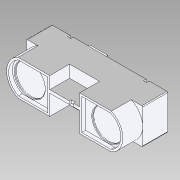
# Autodesk Inventor part: Sharp_2Y0A710
Saved by Autodesk Inventor 2017 (Build 210142000, 142)
## iProperties
Created: 2015-09-16
Part Number: Sharp_2Y0A710
Material: Generic
Document SubType Name: Modeling
Designer: JonathanC
Density: 1 g/cm^3
Appearance: PTFE
Author: JonathanC
Autodesk Inventor part; units mm, degrees
ref_plane "YZ Plane" through (0, 0, 0) normal (1, 0, 0) x (0, 1, 0)
ref_plane "XZ Plane" through (0, 0, 0) normal (0, 1, 0) x (-1, 0, 0)
ref_plane "XY Plane" through (0, 0, 0) normal (0, 0, 1) x (1, 0, 0)
sketch "Sketch1" plane through (0, 0, 0) normal (0, 0, 1) x (1, 0, 0)
  line L0 (0, 0) -> (58.039, 0)
  line L1 (58.039, 0) -> (58.039, 17.653)
  line L2 (58.039, 17.653) -> (0, 17.653)
  line L3 (0, 17.653) -> (0, 0)
  dimension "d0" = 58.039
  dimension "d1" = 17.653
  constraints: 8 end point, 2 parallel, 1 horizontal, 1 perpendicular
  measures "d0" distance of L2.end L1.end
  measures "d1" distance of L1.end L0.end
extrude "Extrusion1" add sketch "Sketch1" along normal blind 12.573
sketch "Sketch2" plane through (0, 0, 0) normal (0, 0, -1) x (-1, 0, 0)
  line L0 (0, 0) -> (-58.039, 0) projected
  line L1 (0, 17.653) -> (0, 0) projected
  line L2 (-58.039, 17.653) -> (0, 17.653) projected
  line L3 (-58.039, 0) -> (-58.039, 17.653) projected
  line L4 (-0.889, 16.764) -> (-0.889, 0.889)
  line L5 (-0.889, 0.889) -> (-57.15, 0.889)
  line L6 (-57.15, 0.889) -> (-57.15, 16.764)
  line L7 (-57.15, 16.764) -> (-0.889, 16.764)
  dimension "d4" = 0.889
  constraints: 8 end point, 3 other
  measures "d4" distance between parallel lines of L2 L7
extrude "Extrusion2" cut sketch "Sketch2" against normal blind 1.778 contours L4 L5 L6 L7
sketch "Sketch3" plane through (0, 0, 0) normal (0, -1, 0) x (1, 0, 0)
  line L0 (0, 0) -> (58.039, 0) projected
  line L1 (58.039, 0) -> (58.039, 12.573) projected
  line L2 (0, 12.573) -> (58.039, 12.573) projected
  line L3 (0, 0) -> (0, 12.573) projected
  line L4 (0, 0) -> (58.039, 0) projected
  line L5 (48.768, 0) -> (47.244, 0)
  line L6 (47.244, 0) -> (47.244, 1.27)
  line L7 (47.244, 1.27) -> (48.768, 1.27)
  line L8 (48.768, 1.27) -> (48.768, 0)
  line L9 (10.795, 0) -> (9.271, 0)
  line L10 (9.271, 0) -> (9.271, 1.27)
  line L11 (9.271, 1.27) -> (10.795, 1.27)
  line L12 (10.795, 1.27) -> (10.795, 0)
  dimension "d7" = 1.524
  dimension "d8" = 1.524
  dimension "d9" = 9.271
  dimension "d10" = 9.271
  dimension "d11" = 1.27
  dimension "d12" = 1.27
  constraints: 16 end point, 4 parallel, 2 horizontal, 2 perpendicular, 2 point on line
  measures "d7" distance of L6.end L7.end
  measures "d8" distance of L10.end L11.end
  measures "d9" distance between parallel lines of L1 L8
  measures "d10" distance between parallel lines of L3 L10
  measures "d11" distance of L11.end L9.start
  measures "d12" distance of L5.end L6.end
extrude "Extrusion3" cut sketch "Sketch3" against normal through all contours L10 L11 L12 L0 | L6 L7 L8 L0
sketch "Sketch4" plane through (0, 0, 12.573) normal (0, 0, 1) x (1, 0, 0)
  line L0 (58.039, 17.653) -> (0, 17.653) projected
  line L1 (0, 0) -> (58.039, 0) projected
  line L2 (5.715, 17.653) -> (21.59, 17.653)
  line L3 (21.59, 17.653) -> (21.59, 0)
  line L4 (21.59, 0) -> (5.715, 0)
  line L5 (5.715, 0) -> (5.715, 17.653)
  line L6 (36.5125, 17.653) -> (52.3875, 17.653)
  line L7 (52.3875, 17.653) -> (52.3875, 0)
  line L8 (52.3875, 0) -> (36.5125, 0)
  line L9 (36.5125, 0) -> (36.5125, 17.653)
  arc A0 (52.3875, 0) -> (52.3875, 17.653) centre (48.429, 8.8265) ccw
  arc A1 (5.715, 17.653) -> (5.715, 0) centre (9.6735, 8.8265) ccw
  line L10 (0, 17.653) -> (0, 0) projected
  line L11 (21.59, 11.557) -> (36.5125, 11.557)
  line L12 (36.5125, 11.557) -> (36.5125, 10.033)
  line L13 (36.5125, 10.033) -> (21.59, 10.033)
  line L14 (21.59, 10.033) -> (21.59, 11.557)
  dimension "d17" = 15.875
  dimension "d18" = 15.875
  dimension "d19" = 21.59
  dimension "d20" = 21.59
  dimension "d21" = 1.524
  dimension "d22" = 6.096
  constraints: 24 end point, 6 parallel, 6 point on line, 4 point on circle, 3 horizontal, 3 perpendicular, 2 centre point, 1 tangent
  measures "d17" distance between parallel lines of L3 L5
  measures "d18" distance between parallel lines of L7 L9
  measures "d19" distance between parallel lines of L10 L3
  measures "d21" distance between parallel lines of L11 L13
  measures "d22" distance between parallel lines of L0 L11
extrude "Extrusion4" add sketch "Sketch4" along normal blind 9.906 contours L7 L1 L9 L0 | A0 L7 | L3 L1 L5 L0 | L9 L13 L3 L11 | L5 A1
sketch "Sketch5" plane through (0, 0, 22.479) normal (0, 0, 1) x (1, 0, 0)
  line L0 (21.59, 10.033) -> (36.5125, 10.033) projected
  line L1 (36.5125, 10.033) -> (36.5125, 0) projected
  line L2 (36.5125, 0) -> (52.3875, 0) projected
  arc A0 (52.3875, 0) -> (52.3875, 17.653) centre (48.429, 8.8265) ccw projected
  line L3 (52.3875, 17.653) -> (36.5125, 17.653) projected
  line L4 (36.5125, 17.653) -> (36.5125, 11.557) projected
  line L5 (36.5125, 11.557) -> (21.59, 11.557) projected
  line L6 (21.59, 11.557) -> (21.59, 17.653) projected
  line L7 (21.59, 17.653) -> (5.715, 17.653) projected
  arc A1 (5.715, 17.653) -> (5.715, 0) centre (9.6735, 8.8265) ccw projected
  line L8 (5.715, 0) -> (21.59, 0) projected
  line L9 (21.59, 0) -> (21.59, 10.033) projected
  line L10 (5.7724, 16.5553) -> (20.4923, 16.5553)
  line L11 (20.4923, 16.5553) -> (20.4923, 9.779)
  line L12 (21.59, 9.779) -> (36.5125, 9.779)
  line L13 (37.5285, 8.6762) -> (37.5285, 16.637)
  line L14 (37.5285, 16.637) -> (52.1638, 16.637)
  arc A2 (52.1638, 1.016) -> (52.1638, 16.637) centre (48.429, 8.8265) ccw
  line L15 (52.1638, 1.016) -> (37.5285, 1.016)
  line L16 (37.5285, 1.016) -> (37.5285, 11.811)
  line L17 (36.5125, 11.811) -> (21.59, 11.811)
  line L18 (20.574, 11.811) -> (20.574, 1.016)
  line L19 (20.574, 1.016) -> (5.9387, 1.016)
  arc A3 (5.7724, 16.5553) -> (5.9387, 1.016) centre (9.6735, 8.8265) ccw
  line L20 (37.5285, 16.637) -> (37.5285, 1.016)
  line L21 (0.889, 0.889) -> (57.15, 0.889) projected
  line L22 (52.1638, 1.016) -> (37.5285, 1.016)
  line L23 (20.4923, 16.5553) -> (20.574, 1.016)
  point P0 (0, 0)
  dimension "d25" = 1.016
  dimension "d26" = 1.016
  constraints: 26 end point, 4 point on circle, 4 point on line, 2 centre point, 1 parallel, 1 perpendicular, 7 other
  measures "d25" distance between parallel lines of L9 L18
  measures "d26" distance between parallel lines of L16 L1
extrude "Extrusion5" cut sketch "Sketch5" against normal blind 1.905 contours L10 L23 L19 A3 | L13 L14 A2 L15 L16
sketch "Sketch6" plane through (0, 0, 20.574) normal (0, 0, 1) x (1, 0, 0)
  line L0 (5.7724, 16.5553) -> (20.4923, 16.5553) projected
  arc A0 (5.7724, 16.5553) -> (5.9387, 1.016) centre (9.6735, 8.8265) ccw projected
  line L1 (20.574, 1.016) -> (5.9387, 1.016) projected
  line L2 (20.4923, 16.5553) -> (20.574, 1.016) projected
  line L3 (37.5285, 1.016) -> (37.5285, 16.637) projected
  line L4 (52.1638, 1.016) -> (37.5285, 1.016) projected
  arc A1 (52.1638, 1.016) -> (52.1638, 16.637) centre (48.429, 8.8265) ccw projected
  line L5 (37.5285, 16.637) -> (52.1638, 16.637) projected
  circle A2 centre (9.6735, 8.8265) radius 7.493
  circle A3 centre (48.429, 8.8265) radius 7.493
  point P0 (0, 0)
  dimension "d29" = 14.986
  dimension "d30" = 14.986
  constraints: 2 centre point, 2 coincident
  measures "d29" diameter of A2
  measures "d30" diameter of A3
extrude "Extrusion6" cut sketch "Sketch6" against normal blind 3.048 contours A2 | A3
ref_plane "Work Plane1" through (58.039, 8.8265, 0) normal (0, -1, 0) x (1, 0, 0)
sketch "Sketch7" plane through (58.039, 8.8265, 0) normal (0, -1, 0) x (1, 0, 0)
  arc A0 (-40.8725, 19.7802) -> (-55.8585, 19.7802) centre (-48.3655, 10.7276) ccw
  line L0 (-36.449, 22.479) -> (-52.324, 22.479) projected
  line L1 (-55.8585, 17.526) -> (-40.8725, 17.526) projected
  line L2 (-55.8585, 20.574) -> (-40.8725, 20.574) projected
  line L3 (-48.3655, 22.479) -> (-48.3655, 17.526)
  line L4 (-55.8585, 17.526) -> (-40.8725, 17.526) projected
  line L5 (-48.3655, 17.526) -> (-55.8585, 17.526)
  line L6 (-55.8585, 17.526) -> (-55.8585, 19.7802)
  point P0 (-58.039, 0)
  dimension "d34" = 0
  dimension "d35" = 0
  dimension "d36" = 0.7937
  constraints: 6 end point, 3 point on circle, 1 centre point, 1 horizontal, 1 horizontal alignment, 1 midpoint, 1 point on line, 1 tangent
  measures "d34" horizontal distance of L2.start L6.end
  measures "d35" horizontal distance of L2.end A0.start
  measures "d36" distance from line of L2 A0.start
revolve "Revolution1" add sketch "Sketch7" angle 360 about axis through (9.6735, 8.8265, 22.479) along (0, 0, -1) picked at (-51.9744, 20.9224) contours L3 L2 A0 | L3 L1 L6 A0 L2
ref_plane "Work Plane2" through (29.0195, 0, 0) normal (1, 0, 0) x (0, 0, -1)
mirror "Mirror1" about plane through (29.0195, 0, 0) normal (1, 0, 0) of "Revolution1"
sketch "Sketch8" plane through (21.59, 10.033, 12.573) normal (0, -1, 0) x (1, 0, 0)
  line L0 (14.9225, 0) -> (0, 0) projected
  line L1 (14.9225, 0) -> (14.9225, 9.906) projected
  line L2 (0, 9.906) -> (14.9225, 9.906) projected
  line L3 (0, 0) -> (0, 9.906) projected
  circle A0 centre (7.4613, 4.953) radius 2.0955
  line L4 (0, 9.906) -> (14.9225, 9.906) projected
  line L5 (9.8425, 9.906) -> (11.8745, 9.906)
  line L6 (11.8745, 9.906) -> (11.8745, 8.89)
  line L7 (11.8745, 8.89) -> (9.8425, 8.89)
  line L8 (9.8425, 8.89) -> (9.8425, 9.906)
  point P0 (-21.59, -12.573)
  dimension "d39" = 4.191
  dimension "d40" = 2.032
  dimension "d41" = 1.016
  dimension "d43" = 5.08
  constraints: 8 end point, 2 parallel, 1 centre point, 1 horizontal, 1 perpendicular, 1 point on line
  measures "d39" diameter of A0
  measures "d40" distance of L6.end L7.end
  measures "d41" distance of L5.end L6.end
  measures "d43" distance between parallel lines of L1 L8
extrude "Extrusion7" cut sketch "Sketch8" against normal blind 1.905 contours L6 L7 L8 L2
sketch "Sketch9" plane through (0, 0, 1.778) normal (0, 0, -1) x (-1, 0, 0)
  line L0 (-25.273, 15.621) -> (-16.383, 15.621)
  line L1 (-16.383, 15.621) -> (-16.383, 12.192)
  line L2 (-16.383, 12.192) -> (-25.273, 12.192)
  line L3 (-25.273, 12.192) -> (-25.273, 15.621)
  line L4 (-47.244, 17.653) -> (-10.795, 17.653) projected
  line L5 (0, 17.653) -> (0, 0) projected
  dimension "d46" = 8.89
  dimension "d47" = 3.429
  dimension "d48" = 2.032
  dimension "d49" = 16.383
  constraints: 8 end point, 2 parallel, 1 horizontal, 1 perpendicular
  measures "d46" distance of L1.end L2.end
  measures "d47" distance of L0.end L1.end
  measures "d48" distance between parallel lines of L4 L0
  measures "d49" distance between parallel lines of L5 L1
extrude "Extrusion8" add sketch "Sketch9" along normal blind 4.572
sketch "Sketch10" plane through (0, 0, -2.794) normal (0, 0, -1) x (-1, 0, 0)
  line L0 (-16.383, 15.621) -> (-25.273, 15.621) projected
  line L1 (-25.273, 15.621) -> (-25.273, 12.192) projected
  line L2 (-25.273, 12.192) -> (-16.383, 12.192) projected
  line L3 (-16.383, 12.192) -> (-16.383, 15.621) projected
  line L4 (-24.892, 15.24) -> (-16.764, 15.24)
  line L5 (-16.764, 15.24) -> (-16.764, 12.573)
  line L6 (-16.764, 12.573) -> (-24.892, 12.573)
  line L7 (-24.892, 12.573) -> (-24.892, 15.24)
  point P0 (0, 0)
  dimension "d52" = 0.381
  constraints: 8 end point, 3 other
  measures "d52" distance between parallel lines of L0 L4
extrude "Extrusion9" cut sketch "Sketch10" against normal blind 4.191 contours L4 L5 L6 L7
sketch "Sketch11" plane through (25.273, 12.192, 1.778) normal (1, 0, 0) x (0, 0, -1)
  line L0 (4.572, 0) -> (4.572, 3.429) projected
  line L1 (4.572, 2.54) -> (3.175, 2.54)
  line L2 (3.175, 2.54) -> (3.175, 1.651)
  line L3 (3.175, 1.651) -> (4.572, 1.651)
  line L4 (4.572, 1.651) -> (4.572, 2.54)
  line L5 (0, 3.429) -> (4.572, 3.429) projected
  line L6 (0, 0) -> (4.572, 0) projected
  point P0 (1.778, -12.192)
  dimension "d56" = 0.889
  dimension "d57" = 1.651
  dimension "d58" = 1.397
  constraints: 8 end point, 2 parallel, 1 horizontal, 1 perpendicular, 1 point on line
  measures "d56" distance between parallel lines of L5 L1
  measures "d57" distance between parallel lines of L6 L3
  measures "d58" distance between parallel lines of L0 L2
extrude "Extrusion10" cut sketch "Sketch11" against normal through all
sketch "Sketch12" plane through (0, 0, 1.397) normal (0, 0, -1) x (-1, 0, 0)
  line L0 (-23.9607, 14.5415) -> (-23.4527, 14.5415)
  line L1 (-23.4527, 14.5415) -> (-23.4527, 14.0335)
  line L2 (-23.4527, 14.0335) -> (-23.9607, 14.0335)
  line L3 (-23.9607, 14.0335) -> (-23.9607, 14.5415)
  line L4 (-22.5213, 14.5415) -> (-22.0133, 14.5415)
  line L5 (-22.0133, 14.5415) -> (-22.0133, 14.0335)
  line L6 (-22.0133, 14.0335) -> (-22.5213, 14.0335)
  line L7 (-22.5213, 14.0335) -> (-22.5213, 14.5415)
  line L8 (-21.082, 14.5415) -> (-20.574, 14.5415)
  line L9 (-20.574, 14.5415) -> (-20.574, 14.0335)
  line L10 (-20.574, 14.0335) -> (-21.082, 14.0335)
  line L11 (-21.082, 14.0335) -> (-21.082, 14.5415)
  line L12 (-19.6427, 14.5415) -> (-19.1347, 14.5415)
  line L13 (-19.1347, 14.5415) -> (-19.1347, 14.0335)
  line L14 (-19.1347, 14.0335) -> (-19.6427, 14.0335)
  line L15 (-19.6427, 14.0335) -> (-19.6427, 14.5415)
  line L16 (-18.2033, 14.5415) -> (-17.6953, 14.5415)
  line L17 (-17.6953, 14.5415) -> (-17.6953, 14.0335)
  line L18 (-17.6953, 14.0335) -> (-18.2033, 14.0335)
  line L19 (-18.2033, 14.0335) -> (-18.2033, 14.5415)
  line L20 (-24.892, 14.732) -> (-24.892, 15.24) projected
  line L21 (-16.764, 15.24) -> (-16.764, 14.732) projected
  line L22 (-25.273, 14.732) -> (-24.892, 14.732) projected
  line L23 (-24.892, 13.843) -> (-25.273, 13.843) projected
  line L24 (-24.892, 14.732) -> (-24.892, 13.843) projected
  line L25 (-16.764, 13.843) -> (-16.764, 14.732) projected
  point P0 (0, 0)
  dimension "d61" = 0.508
  dimension "d62" = 0.508
  dimension "d63" = 0.9313
  dimension "d64" = 0.9313
  dimension "d65" = 0.9313
  dimension "d66" = 0.9313
  dimension "d67" = 0.9313
  dimension "d68" = 0.9313
  dimension "d69" = 0.1905
  dimension "d70" = 0.1905
  dimension "d72" = 0.9313
  constraints: 40 end point, 10 parallel, 8 equal length, 5 horizontal, 5 perpendicular, 3 point on line, 1 collinear
  measures "d61" distance of L0.start L0.end
  measures "d62" distance of L2.end L0.start
  measures "d63" distance between parallel lines of L7 L1
  measures "d64" distance between parallel lines of L11 L5
  measures "d65" distance between parallel lines of L15 L9
  measures "d66" distance between parallel lines of L19 L13
  measures "d67" distance between parallel lines of L20 L3
  measures "d68" distance between parallel lines of L21 L17
  measures "d69" distance between parallel lines of L22 L0
  measures "d70" distance between parallel lines of L23 L2
  measures "d72" distance between parallel lines of L25 L17
extrude "Extrusion11" add sketch "Sketch12" along normal blind 3.81
chamfer "Chamfer1" distance 0.2646 angle 45 2 edges at (2.1805, 8.8265, 20.574) (40.936, 8.8265, 20.574)
fillet "Fillet1" radius 0.3969 4 edges at (58.039, 17.653, 6.2865) (58.039, 0, 6.2865) (0, 17.653, 6.2865) (0, 0, 6.2865)
equation "\"d61\" = d62"
equation "\"d63\" = d67"
equation "\"d64\" = d63"
equation "\"d65\" = d64"
equation "\"d66\" = d65"
equation "\"d67\" = d72"
equation "\"d69\" = d70"
body "Solid1"
